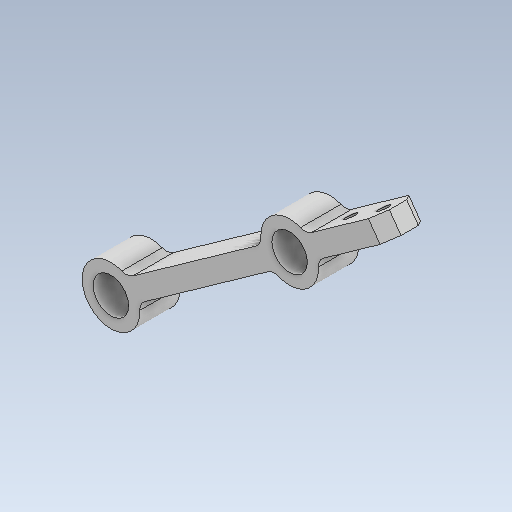
# Autodesk Inventor part: leg_link_1
Saved by Autodesk Inventor 2020 (Build 240168000, 168)
## iProperties
Created: 2020-12-12
Part Number: leg_link_1
Material: Generic
Document SubType Name: Modeling
Designer: Shuang Peng
Density: 1 g/cm^3
Appearance: Default
Author: Shuang Peng
Autodesk Inventor part; units mm, degrees
ref_plane "YZ Plane" through (0, 0, 0) normal (1, 0, 0) x (0, 1, 0)
ref_plane "XZ Plane" through (0, 0, 0) normal (0, 1, 0) x (-1, 0, 0)
ref_plane "XY Plane" through (0, 0, 0) normal (0, 0, 1) x (1, 0, 0)
sketch "Sketch1" plane through (0, 0, 0) normal (0, 0, 1) x (1, 0, 0)
  line L0 (-49.6346, 71.1042) -> (-18.6575, 93.1137)
  circle A0 centre (-49.6346, 71.1042) radius 5
  circle A1 centre (-18.6575, 93.1137) radius 5
  circle A2 centre (-49.6346, 71.1042) radius 3.075
  circle A3 centre (-18.6575, 93.1137) radius 3.075
  line L1 (-49.6346, 71.1042) -> (-18.6575, 93.1137) construction
  line L2 (-48.621, 69.6776) -> (-17.6439, 91.6871)
  line L3 (-19.6711, 94.5403) -> (-50.6482, 72.5308)
  arc A4 (-50.6482, 72.5308) -> (-48.621, 69.6776) centre (-49.6346, 71.1042) ccw
  arc A5 (-17.6439, 91.6871) -> (-19.6711, 94.5403) centre (-18.6575, 93.1137) ccw
  line L4 (-18.6575, 93.1137) -> (-2.3537, 104.6976) construction
  line L5 (-17.6439, 91.6871) -> (-1.3401, 103.271)
  line L6 (-3.3673, 106.1242) -> (-19.6711, 94.5403)
  arc A6 (-19.6711, 94.5403) -> (-17.6439, 91.6871) centre (-18.6575, 93.1137) ccw
  arc A7 (-1.3401, 103.271) -> (-3.3673, 106.1242) centre (-2.3537, 104.6976) ccw
  line L7 (-2.3537, 104.6976) -> (-3.3673, 106.1242)
  line L8 (-2.3537, 104.6976) -> (-1.3401, 103.271)
  point P0 (0, 0)
  point P1 (-34.1461, 82.109)
  point P2 (-10.5056, 98.9057)
  point P3 (-44.8029, 72.3905)
  point P4 (-21.462, 88.9743)
  point P5 (-13.8258, 94.3999)
  point P6 (-15.8529, 97.2531)
  point P7 (-23.4892, 91.8275)
  point P8 (-46.8301, 75.2436)
  dimension "d0" = 10
  dimension "d1" = 10
  dimension "d2" = 6.15
  dimension "d3" = 6.15
  dimension "d4" = 3.5
  dimension "d5" = 20
  dimension "d6" = 3.5
  constraints: 22 end point, 8 centre point, 8 point on circle, 8 tangent, 4 coincident, 2 collinear, 2 midpoint, 2 parallel
  measures "d0" diameter of A0
  measures "d1" diameter of A1
  measures "d2" diameter of A2
  measures "d3" diameter of A3
  measures "d4" diameter of A5
  measures "d5" distance of L1.end L4.end
  measures "d6" diameter of A7
extrude "Extrusion1" add sketch "Sketch1" along normal mid plane 7 contours A2 L3 A0 L0 | L0 A0 L2 A2 | A0 L3 A1 L0 | L0 A1 L2 A0 | L2 A0 L3 A2 | A1 L3 A3 L0 | L0 A3 L2 A1 | A1 L6 A3 L3 | L2 A3 L5 A1 | L6 L7 L8 L5 A1 | A1 L5 A3 L6
sketch "Sketch2" plane through (-1.3401, 103.271, -3.5) normal (0.5791965, -0.8151879, 0) x (0.8151879, 0.5791965, 0)
  line L0 (0, 0) -> (0, 7) projected
  line L1 (-15.3163, 7) -> (0, 7) projected
  line L2 (-15.3163, 0) -> (-15.3163, 7) projected
  line L3 (0, 0) -> (-15.3163, 0) projected
  line L4 (0, 0) -> (0, 7) projected
  line L5 (0, 3.5) -> (-8, 3.5)
  line L6 (-8, 3.5) -> (-3, 3.5)
  circle A0 centre (-3, 3.5) radius 1
  line L7 (-8, 3.5) -> (-10, 3.5)
  circle A1 centre (-10, 3.5) radius 1
  point P0 (-58.7218, 3.5)
  dimension "d9" = 8
  dimension "d10" = 5
  dimension "d11" = 2
  dimension "d12" = 2
  dimension "d13" = 2
  constraints: 6 end point, 2 centre point, 2 coincident, 2 horizontal, 1 midpoint, 1 point on line
  measures "d9" distance of L5.start L5.end
  measures "d10" distance of L5.end L6.end
  measures "d11" diameter of A0
  measures "d12" distance of L5.end L7.end
  measures "d13" diameter of A1
extrude "Extrusion2" cut sketch "Sketch2" against normal blind 5 contours A0 L5 | L5 A0 | A1
fillet "Fillet1" radius 2 6 edges at (-46.8301, 75.2436, 0) (-44.8029, 72.3905, 0) (-21.462, 88.9743, 0) (-13.8258, 94.3999, 0) (-15.8529, 97.2531, 0) (-23.4892, 91.8275, 0)
chamfer "Chamfer1" distance 2 angle 45 2 edges at (-2.3537, 104.6976, 3.5) (-2.3537, 104.6976, -3.5)
body "Solid1"
